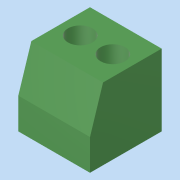
# Autodesk Inventor part: connector
Saved by Autodesk Inventor 2017 (Build 210142000, 142)
## iProperties
Created: 2017-01-25
Part Number: connector
Material: Generic
Document SubType Name: Modeling
Designer: techn
Density: 1 g/cm^3
Appearance: Smooth - Dark Forest Green
Author: techn
Autodesk Inventor part; units mm, degrees
ref_plane "YZ Plane" through (0, 0, 0) normal (1, 0, 0) x (0, 1, 0)
ref_plane "XZ Plane" through (0, 0, 0) normal (0, 1, 0) x (-1, 0, 0)
ref_plane "XY Plane" through (0, 0, 0) normal (0, 0, 1) x (1, 0, 0)
sketch "Sketch1" plane through (0, 0, 0) normal (0, 1, 0) x (-1, 0, 0)
  line L0 (0, 0) -> (5.588, 0)
  line L1 (5.588, 0) -> (5.588, -5.588)
  line L2 (5.588, -5.588) -> (0, -5.588)
  line L3 (0, -5.588) -> (0, 0)
  dimension "d0" = 5.588
  dimension "d1" = 5.588
  constraints: 8 end point, 2 parallel, 1 horizontal, 1 perpendicular
  measures "d0" distance of L1.end L2.end
  measures "d1" distance of L0.end L1.end
extrude "Extrusion1" add sketch "Sketch1" along normal blind 5.588
chamfer "Chamfer1" distance 1.016 distance2 3.175 1 edges at (-2.794, 5.588, 0) measured on face at (-1.8627, 5.588, -1.8627)
sketch "Sketch2" plane through (0, 5.588, 0) normal (0, 1, 0) x (1, 0, 0)
  line L0 (0, 1.016) -> (-5.588, 1.016) projected
  line L1 (0, 1.016) -> (0, 5.588) projected
  line L2 (0, 5.588) -> (-5.588, 5.588) projected
  line L3 (-5.588, 5.588) -> (-5.588, 1.016) projected
  circle A0 centre (-4.064, 3.302) radius 0.9525
  circle A1 centre (-1.524, 3.302) radius 0.9525
  point P0 (0, 0)
  dimension "d7" = 1.905
  dimension "d8" = 1.905
  dimension "d9" = 1.524
  dimension "d10" = 1.524
  constraints: 2 centre point
  measures "d7" diameter of A0
  measures "d8" diameter of A1
  measures "d9" distance from line of A0.centre L3
  measures "d10" distance from line of L1 A1.centre
extrude "Extrusion2" cut sketch "Sketch2" against normal blind 2.54 contours A0 | A1
body "Solid1"
